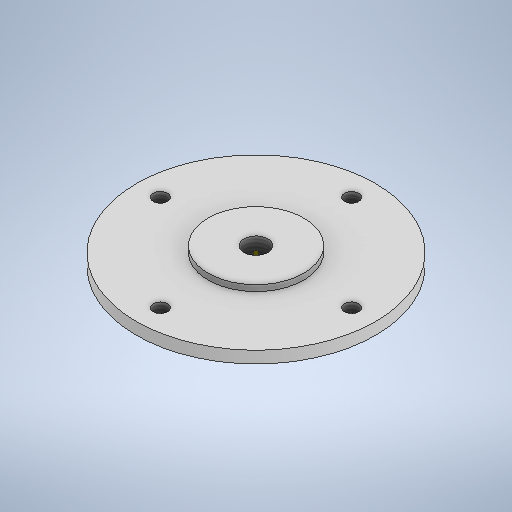
# Autodesk Inventor part: płytka
Saved by Autodesk Inventor 2025.2 (Build 292293000, 293)
## iProperties
Created: 2025-03-15
Part Number: płytka
Material: Ogólny
Document SubType Name: Modeling
Designer: barte
Density: 1 g/cm^3
Appearance: Domyślna
Author: barte
Autodesk Inventor part; units mm, degrees
ref_plane "YZ Plane" through (0, 0, 0) normal (1, 0, 0) x (0, 1, 0)
ref_plane "XZ Plane" through (0, 0, 0) normal (0, 1, 0) x (-1, 0, 0)
ref_plane "XY Plane" through (0, 0, 0) normal (0, 0, 1) x (1, 0, 0)
sketch "Szkic1" plane through (0, 0, 0) normal (0, 1, 0) x (-1, 0, 0)
  circle A0 centre (0, 0) radius 50
  circle A1 centre (0, 40) radius 3
  circle A2 centre (0, -40) radius 3
  circle A3 centre (40, 0) radius 3
  circle A4 centre (-40, 0) radius 3
  circle A5 centre (0, 0) radius 20
  dimension "d0" = 100
  dimension "d1" = 6
  dimension "d2" = 6
  dimension "d3" = 6
  dimension "d4" = 6
  dimension "d5" = 40
  dimension "d6" = 80
  dimension "d7" = 40
  dimension "d8" = 80
  dimension "d9" = 40
  constraints: 6 centre point, 2 coincident
  measures "d0" diameter of A0
  measures "d1" diameter of A1
  measures "d2" diameter of A2
  measures "d3" diameter of A3
  measures "d4" diameter of A4
  measures "d5" distance of point (0, 0) A1.centre
  measures "d6" distance of A2.centre A1.centre
  measures "d7" distance of point (0, 0) A3.centre
  measures "d8" distance of A4.centre A3.centre
  measures "d9" diameter of A5
extrude "Wyciągnięcie proste1" add sketch "Szkic1" along normal blind 5
sketch "Szkic2" plane through (0, 5, 0) normal (0, 1, 0) x (1, 0, 0)
  point P0 (0, 0)
sketch "Szkic3" plane through (0, 5, 0) normal (0, 1, 0) x (1, 0, 0)
  circle A0 centre (0, 0) radius 20
  circle A1 centre (0, 0) radius 5
  dimension "d12" = 40
  dimension "d13" = 10
  constraints: 2 centre point, 2 coincident
  measures "d12" diameter of A0
  measures "d13" diameter of A1
extrude "Wyciągnięcie proste2" add sketch "Szkic3" along normal blind 2.5 and the other way blind 5
thread "Gwint1" size "M10x1.5" class "6H" standard "ANSI Metric M Profile" length 100
thread "Gwint2" size "M10x1.5" class "6H" standard "ANSI Metric M Profile" length 100
thread "Gwint3" size "M10x1.5" class "6H" standard "ANSI Metric M Profile" length 100
thread "Gwint4" size "M10x1.5" class "6H" standard "ANSI Metric M Profile" length 100
thread "Gwint5" size "M10x1.5" class "6H" standard "ANSI Metric M Profile" length 31.37
